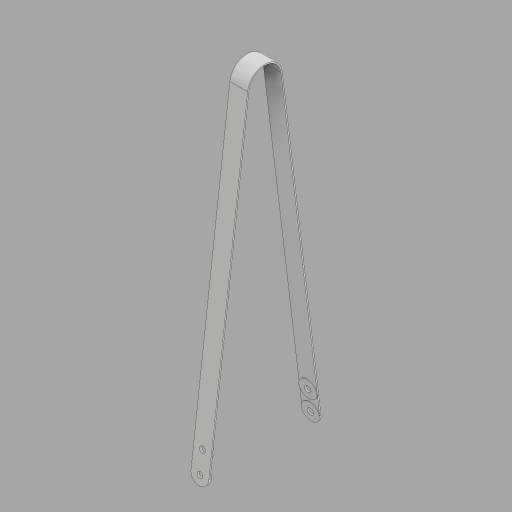
# Autodesk Inventor part: szalag5
Saved by Autodesk Inventor 2023 (Build 270158000, 158)
## iProperties
Created: 2022-11-18
Part Number: szalag5
Material: Generic
Document SubType Name: Modeling
Designer: gd1
Density: 1 g/cm^3
Appearance: Default
Author: gd1
Autodesk Inventor part; units mm, degrees
ref_plane "YZ Plane" through (0, 0, 0) normal (1, 0, 0) x (0, 1, 0)
ref_plane "XZ Plane" through (0, 0, 0) normal (0, 1, 0) x (-1, 0, 0)
ref_plane "XY Plane" through (0, 0, 0) normal (0, 0, 1) x (1, 0, 0)
sketch "Sketch1" plane through (0, 0, 0) normal (1, 0, 0) x (0, 1, 0)
  circle A0 centre (0, 0) radius 14.612
  line L0 (0, 0) -> (-254.37, 0)
  line L1 (0, 0) -> (254.37, 0) construction
  line L2 (-271.87, -50) -> (-236.87, -50)
  line L3 (-236.87, -50) -> (-236.87, 50) construction
  line L4 (-236.87, 50) -> (-271.87, 50)
  line L5 (-271.87, 50) -> (-271.87, -50) construction
  line L6 (-271.87, -50) -> (-236.87, 50) construction
  line L7 (-236.87, -50) -> (-271.87, 50) construction
  line L8 (-271.87, 50) -> (-271.87, 48)
  line L9 (-271.87, 48) -> (1.775368, 14.503745)
  circle A1 centre (0, 0) radius 13.612
  line L10 (-271.87, 48) -> (-271.87, 47)
  line L11 (-271.87, 47) -> (1.65423, 13.511109)
  line L12 (-271.87, -48) -> (1.775368, -14.503745)
  line L13 (-271.87, -47) -> (1.65423, -13.511109)
  line L14 (-271.87, -48) -> (-271.87, -47)
  point P0 (1.65423, -13.511109)
  point P1 (1.775368, -14.503745)
  dimension "d0" = 29.224
  dimension "d6" = 1
  dimension "d1" = 254.37
  dimension "d2" = 180
  dimension "d3" = 35
  dimension "d4" = 100
  dimension "d5" = 2
  dimension "d7" = 1
  constraints: 30 end point, 4 symmetric about line, 3 horizontal, 2 collinear, 2 midpoint, 2 parallel, 2 point on line, 1 coincident, 1 perpendicular, 8 other
  measures "d1" distance of L0.start L0.end
  measures "d2" angle of L0 L1
  measures "d3" distance of L4.end L3.end
  measures "d4" distance of L3.end L2.end
  measures "d5" distance of L4.end L8.end
  measures "d7" distance of L8.end L10.end
extrude "Extrusion1" add sketch "Sketch1" along normal blind 15 contours A0 L13 A1 L11 | A0 L11 L10 L9 | L12 L14 L13 A0
sketch "Sketch2" plane through (15, 1.65423, 13.511109) normal (0, -0.1215273, -0.9925881) x (-1, 0, 0)
  line L0 (15, -275.688235) -> (0, -275.688235)
  line L1 (15, -275.688235) -> (0, -275.688235)
  line L2 (0, -275.688235) -> (0, -260.688235)
  line L3 (0, -260.688235) -> (15, -260.688235)
  line L4 (15, -260.688235) -> (15, -275.688235)
  line L5 (15, -0.000393) -> (15, -275.688235)
  line L6 (0, -260.688235) -> (15, -260.688235)
  line L7 (15, -260.688235) -> (15, -258.188235)
  line L8 (15, -258.188235) -> (0, -258.188235)
  line L9 (0, -258.188235) -> (0, -260.688235)
  line L10 (15, -258.188235) -> (0, -258.188235)
  line L11 (0, -258.188235) -> (0, -243.188235)
  line L12 (0, -243.188235) -> (15, -243.188235)
  line L13 (15, -243.188235) -> (15, -258.188235)
  circle A0 centre (7.5, -250.688235) radius 7.5
  circle A1 centre (7.5, -268.188235) radius 7.5
  circle A2 centre (7.5, -268.188235) radius 2.382127
  circle A3 centre (7.5, -250.688235) radius 2.382127
  point P0 (15, 0)
  point P1 (15, -268.188235)
  point P2 (7.5, -275.688235)
  point P3 (0, -268.188235)
  point P4 (0, -275.688235)
  dimension "d10" = 15
  dimension "d11" = 15
  dimension "d12" = 2.5
  dimension "d13" = 15
  dimension "d14" = 15
  constraints: 24 end point, 6 parallel, 4 centre point, 3 horizontal, 3 perpendicular, 2 coincident, 1 point on line, 1 tangent
  measures "d10" distance of L2.end L3.end
  measures "d11" distance of L1.end L2.end
  measures "d12" distance of L7.end L6.end
  measures "d13" distance of L11.end L12.end
  measures "d14" distance of L10.end L11.end
extrude "Extrusion2" add sketch "Sketch2" along normal blind 1 contours A1 | A0 | A2 | A3
extrude "Extrusion3" cut sketch "Sketch2" along normal mid plane 2 contours A2 | A3
extrude "Extrusion4" cut sketch "Sketch2" along normal mid plane 2 contours L0 A1 L4 | L0 L2 A1
sketch "Sketch3" plane through (0, -271.87, -47) normal (0, -0.1215273, 0.9925881) x (1, 0, 0)
  line L0 (0, -0.121527) -> (15, -0.121527)
  line L1 (0, -0.121527) -> (15, -0.121527)
  line L2 (15, -0.121527) -> (15, 14.878473)
  line L3 (15, 14.878473) -> (0, 14.878473)
  line L4 (0, 14.878473) -> (0, -0.121527)
  line L5 (0, -0.121527) -> (0, 275.566315)
  line L6 (15, 14.878473) -> (0, 14.878473)
  line L7 (0, 14.878473) -> (0, 17.378473)
  line L8 (0, 17.378473) -> (15, 17.378473)
  line L9 (15, 17.378473) -> (15, 14.878473)
  line L10 (0, 17.378473) -> (15, 17.378473)
  line L11 (15, 17.378473) -> (15, 33.595058)
  line L12 (15, 33.595058) -> (0, 33.595058)
  line L13 (0, 33.595058) -> (0, 17.378473)
  circle A0 centre (7.5, 7.378473) radius 7.5
  circle A1 centre (7.5, 24.878473) radius 7.5
  circle A2 centre (7.5, 7.378473) radius 2.75
  circle A3 centre (7.5, 24.878473) radius 2.75
  point P0 (0, 275.566708)
  point P1 (15, 7.378473)
  point P2 (7.5, -0.121527)
  point P3 (0, 7.378473)
  dimension "d21" = 15
  dimension "d22" = 15
  dimension "d23" = 2.5
  dimension "d24" = 15
  dimension "d27" = 5.5
  dimension "d33" = 5.5
  dimension "d34" = 15
  constraints: 24 end point, 6 parallel, 4 centre point, 3 horizontal, 3 perpendicular, 2 coincident, 2 tangent, 1 point on line
  measures "d21" distance of L3.end L2.end
  measures "d22" distance of L2.end L1.end
  measures "d23" distance of L6.end L7.end
  measures "d24" distance of L12.end L11.end
  measures "d27" diameter of A2
  measures "d33" diameter of A3
  measures "d34" diameter of A1
extrude "Extrusion5" add sketch "Sketch3" along normal mid plane 1 contours A0 | A1 | A2 | A3
extrude "Extrusion6" cut sketch "Sketch3" along normal mid plane 2 contours A2 | A3
extrude "Extrusion7" cut sketch "Sketch3" along normal mid plane 2 contours L4 A0 L0 | A0 L2 L0
body "Solid1"
